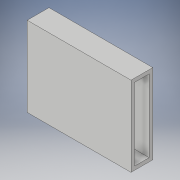
# Autodesk Inventor part: Marcus' Case
Saved by Autodesk Inventor 2018 (Build 220112000, 112)
## iProperties
Created: 2019-09-03
Part Number: Marcus' Case
Material: Generic
Document SubType Name: Modeling
Designer: 871357
Density: 1 g/cm^3
Appearance: Default
Author: 871357
Autodesk Inventor part; units mm, degrees
ref_plane "YZ Plane" through (0, 0, 0) normal (1, 0, 0) x (0, 1, 0)
ref_plane "XZ Plane" through (0, 0, 0) normal (0, 1, 0) x (-1, 0, 0)
ref_plane "XY Plane" through (0, 0, 0) normal (0, 0, 1) x (1, 0, 0)
sketch "Sketch1" plane through (0, 0, 0) normal (0, 0, 1) x (1, 0, 0)
  line L0 (0, 0) -> (-87.63, 0)
  line L1 (-87.63, 0) -> (-87.63, 63.5)
  line L2 (-87.63, 63.5) -> (0, 63.5)
  line L3 (0, 63.5) -> (0, 0)
  dimension "d0" = 87.63
  dimension "d1" = 63.5
  constraints: 8 end point, 2 parallel, 1 horizontal, 1 perpendicular
  measures "d0" distance of L1.end L2.end
  measures "d1" distance of L0.end L1.end
sketch "Sketch2" plane through (0, 0, 0) normal (0, 0, 1) x (1, 0, 0)
  line L0 (0, -3.175) -> (-90.805, -3.175)
  line L1 (-90.805, -3.175) -> (-90.805, 66.675)
  line L2 (-90.805, 66.675) -> (0, 66.675)
  line L3 (0, 66.675) -> (0, -3.175)
  line L4 (-87.63, 63.5) -> (0, 63.5) projected
  point P0 (0, 0)
  dimension "d2" = 3.175
  dimension "d3" = 3.175
  dimension "d4" = 66.675
  dimension "d6" = 0
  constraints: 8 end point, 2 parallel, 1 horizontal, 1 perpendicular
  measures "d2" distance between parallel lines of L4 L2
  measures "d3" distance from line of L4.start L1
  measures "d4" distance between parallel lines of L4 L0
  measures "d6" distance from line of L4.end L3
extrude "Extrusion1" add sketch "Sketch2" along normal mid plane 19.05
extrude "Extrusion2" cut sketch "Sketch1" along normal mid plane 12.7
body "Solid1"
